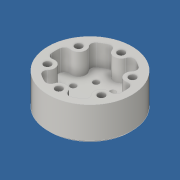
# Autodesk Inventor part: GripperMount
Saved by Autodesk Inventor 2016 (Build 200138000, 138)
## iProperties
Created: 2015-09-10
Part Number: GripperMount
Material: ABS-Kunststoff
Document SubType Name: Modeling
Designer: 4ndreas
Density: 1.06 g/cm^3
Appearance: Glatt - weiß
Mass: 7.57349 g
Surface Area: 55.223 cm^2
Volume: 7.1448 cm^3
Author: 4ndreas
Autodesk Inventor part; units mm, degrees
ref_plane "YZ Plane" through (0, 0, 0) normal (1, 0, 0) x (0, 1, 0)
ref_plane "XZ Plane" through (0, 0, 0) normal (0, 1, 0) x (-1, 0, 0)
sketch "Skizze1" plane through (0, 0, 0) normal (0, 0, 1) x (1, 0, 0)
  circle A0 centre (0, 0) radius 17.5
  dimension "d0" = 35
  constraints: 1 centre point, 1 coincident
  measures "d0" diameter of A0
extrude "Extrusion1" add sketch "Skizze1" along normal blind 14
sketch "Skizze2" plane through (0, 0, 0) normal (0, 0, -1) x (-1, 0, 0)
  circle A0 centre (0, 0) radius 9.5
  dimension "d3" = 19
  constraints: 1 centre point, 1 coincident
  measures "d3" diameter of A0
extrude "Extrusion2" cut sketch "Skizze2" against normal blind 2
ref_plane "Arbeitsebene2" through (0, 0, 14) normal (0, 0, 1) x (1, 0, 0)
sketch "Skizze4" plane through (0, 0, 14) normal (0, 0, 1) x (1, 0, 0)
  circle A0 centre (0, 0) radius 9.5 construction
  circle A1 centre (0, 0) radius 17.5 projected
  circle A2 centre (0, 0) radius 14.5
  dimension "d9" = 3
  constraints: 1 centre point, 1 coincident
  measures "d9" radial gap between concentric circles of A2 A1
extrude "Extrusion4" cut sketch "Skizze4" against normal blind 9 contours A2
chamfer "Fase1" distance 1 angle 45 1 edges at (-17.5, 0, 0)
sketch "Skizze5" plane through (0, 0, 5) normal (0, 0, 1) x (1, 0, 0)
  circle A0 centre (0, 0) radius 9 projected
  circle A1 centre (6.8228, 1.5652) radius 0.85 projected
  circle A2 centre (6.6913, -2.0559) radius 0.85 projected
  circle A3 centre (4.7669, -5.1261) radius 0.85 projected
  circle A4 centre (1.5652, -6.8228) radius 0.85 projected
  circle A5 centre (-2.0559, -6.6913) radius 0.85 projected
  circle A6 centre (-5.1261, -4.7669) radius 0.85 projected
  circle A7 centre (-6.8228, -1.5652) radius 0.85 projected
  circle A8 centre (-6.6913, 2.0559) radius 0.85 projected
  circle A9 centre (-4.7669, 5.1261) radius 0.85 projected
  circle A10 centre (-1.5652, 6.8228) radius 0.85 projected
  circle A11 centre (2.0559, 6.6913) radius 0.85 projected
  circle A12 centre (5.1261, 4.7669) radius 0.85 projected
  circle A13 centre (0, 0) radius 4 projected
  line L0 (0, 0) -> (-4.7669, 5.1261) construction
  point P0 (0, 0)
  dimension "d18" = 7
  constraints: 2 end point
  measures "d18" distance of L0.start L0.end
extrude "Extrusion5" [suppressed]
sketch "Skizze6" plane through (0, 0, 14) normal (0, 0, 1) x (1, 0, 0)
  circle A0 centre (0, 0) radius 14.5 projected
  circle A1 centre (0, 0) radius 17.5 projected
sketch "Skizze7" plane through (0, 0, 5) normal (0, 0, 1) x (1, 0, 0)
  circle A0 centre (0, 0) radius 7 construction
  line L0 (3.5, 6.0622) -> (7, 0) construction
  line L1 (7, 0) -> (3.5, -6.0622) construction
  line L2 (3.5, -6.0622) -> (-3.5, -6.0622) construction
  line L3 (-3.5, -6.0622) -> (-7, 0) construction
  line L4 (-7, 0) -> (-3.5, 6.0622) construction
  line L5 (-3.5, 6.0622) -> (3.5, 6.0622) construction
  dimension "d19" = 14
  constraints: 12 end point, 2 coincident, 1 horizontal, 16 other
hole "Bohrung1" at (-3.5, 6.0622, 5) at (-7, 0, 5) at (-3.5, -6.0622, 5) at (3.5, -6.0622, 5) at (7, 0, 5) at (3.5, 6.0622, 5) direction (0, 0, -1) diameter 2.5 end through all
sketch "Skizze8" plane through (0, 0, 14) normal (0, 0, 1) x (1, 0, 0)
  circle A0 centre (0, 13) radius 3
  circle A1 centre (0, 0) radius 14.5 projected
  circle A2 centre (0, 0) radius 17.5 projected
  circle A3 centre (0, 0) radius 14.5 projected
  line L0 (0, 0) -> (0, 13) construction
  line L1 (-3, 13) -> (-3, 14.1863)
  line L2 (3, 13) -> (3, 14.1863)
  dimension "d27" = 6
  dimension "d38" = 13
  constraints: 6 end point, 6 point on circle, 2 parallel, 2 tangent, 1 centre point, 1 vertical
  measures "d27" diameter of A0
  measures "d38" distance of L0.start L0.end
extrude "Extrusion6" add sketch "Skizze8" against normal up to surface (9 mm away) contours A0 A1 | L1 A1 A0 | A0 A1 L2 picked at (0.1205, 12.988)
fillet "Rundung1" radius 2 2 edges at (-3, 14.1863, 9.5) (3, 14.1863, 9.5)
sketch "Skizze9" plane through (0, 0, 14) normal (0, 0, 1) x (1, 0, 0)
  arc A0 (5.5501, 13.3958) -> (2.8707, 12.1288) centre (4.7846, 11.5481) ccw projected
  arc A1 (-5.5501, 13.3958) -> (5.5501, 13.3958) centre (0, 0) ccw projected
  arc A2 (-2.8707, 12.1288) -> (-5.5501, 13.3958) centre (-4.7846, 11.5481) ccw projected
  arc A3 (-2.8707, 12.1288) -> (2.8707, 12.1288) centre (0, 13) ccw projected
  circle A4 centre (0, 0) radius 17.5 projected
hole "Bohrung2" at (0, 13, 14) direction (0, 0, -1) diameter 3 end through all
sketch "Skizze10" plane through (0, 0, 0) normal (0, 0, -1) x (-1, 0, 0)
  circle A0 centre (0, 13) radius 1.5 projected
  circle A1 centre (0, 0) radius 9.5 projected
  circle A2 centre (0, 0) radius 16.5 projected
  line L0 (2.8868, 13) -> (1.4434, 10.5)
  line L1 (1.4434, 10.5) -> (-1.4434, 10.5)
  line L2 (-1.4434, 10.5) -> (-2.8868, 13)
  line L3 (-2.8868, 13) -> (-1.4434, 15.5)
  line L4 (-1.4434, 15.5) -> (1.4434, 15.5)
  line L5 (1.4434, 15.5) -> (2.8868, 13)
  dimension "d39" = 5
  dimension "d45" = 40
  constraints: 12 end point, 1 coincident, 1 horizontal, 13 other
  measures "d39" distance between parallel lines of L1 L4
extrude "Extrusion7" cut sketch "Skizze10" against normal blind 5 contours A0 | L0 L1 L2 L3 L4 L5
pattern_circular "Runde Anordnung1" count 6 over 360 about axis through (0, 0, 14) along (0, 0, -1) of "Bohrung2", "Extrusion6", "Rundung1", "Extrusion7"
